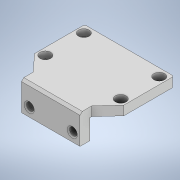
# Autodesk Inventor part: Крышка-6
Saved by Autodesk Inventor 2022 (Build 260153000, 153)
## iProperties
Created: 2021-12-03
Part Number: Крышка-6
Material: Типовые
Document SubType Name: Modeling
Designer: Украинцев
Density: 1 g/cm^3
Appearance: По умолчанию
Author: Украинцев
Autodesk Inventor part; units mm, degrees
ref_plane "YZ Plane" through (0, 0, 0) normal (1, 0, 0) x (0, 1, 0)
ref_plane "XZ Plane" through (0, 0, 0) normal (0, 1, 0) x (-1, 0, 0)
ref_plane "XY Plane" through (0, 0, 0) normal (0, 0, 1) x (1, 0, 0)
sketch "Эскиз1" plane through (0, 0, 0) normal (0, 1, 0) x (-1, 0, 0)
  line L0 (0, 0) -> (58, 0)
  line L1 (58, 0) -> (58, 65)
  line L2 (58, 65) -> (38, 86.8785)
  line L3 (0, 0) -> (0, 102)
  line L4 (0, 102) -> (38, 102)
  line L5 (38, 102) -> (38, 86.8785)
  line L6 (0, 0) -> (49, 0)
  line L7 (49, 0) -> (49, 10)
  line L8 (49, 10) -> (49, 60)
  dimension "d8" = 58
  dimension "d9" = 65
  dimension "d10" = 102
  dimension "d11" = 38
  dimension "d12" = 49
  dimension "d13" = 10
  dimension "d14" = 50
  constraints: 18 end point, 4 perpendicular, 2 coincident, 2 point on line, 1 horizontal, 1 vertical
  measures "d8" distance of L0.start L0.end
  measures "d9" distance of L0.end L1.end
  measures "d10" distance of L0.start L3.end
  measures "d11" distance of L3.end L4.end
  measures "d12" distance of L0.start L6.end
  measures "d13" distance of L6.end L7.end
  measures "d14" distance of L7.end L8.end
extrude "Выдавливание1" add sketch "Эскиз1" along normal blind 12
sketch "Эскиз3" plane through (0, 12, 0) normal (0, 1, 0) x (1, 0, 0)
  line L0 (-38, -102) -> (0, -102) projected
  line L1 (-38, -102) -> (-38, -89)
  line L2 (-38, -86.8785) -> (-38, -102) projected
  line L3 (-38, -89) -> (0, -89)
  line L4 (0, -89) -> (0, -102)
  point P0 (0, 0)
  dimension "d17" = 13
  constraints: 6 end point, 1 perpendicular, 1 point on line, 1 vertical
  measures "d17" distance of L0.start L1.end
extrude "Выдавливание2" add sketch "Эскиз3" against normal blind 38
sketch "Эскиз4" plane through (0, 12, 0) normal (0, 1, 0) x (1, 0, 0)
  line L0 (0, 0) -> (-58, 0) projected
  line L1 (0, 0) -> (-49, 0)
  line L2 (-49, 0) -> (-49, -10)
  line L3 (-49, -10) -> (-49, -60)
  dimension "d20" = 49
  dimension "d21" = 10
  dimension "d22" = 50
  constraints: 6 end point, 2 coincident, 2 point on line, 1 perpendicular
  measures "d20" distance of L0.start L1.end
  measures "d21" distance of L1.end L2.end
  measures "d22" distance of L2.end L3.end
hole "Отверстие1" at (-49, 12, 60) at (-49, 12, 10) direction (0, -1, 0) diameter 9 end through all counterbore diameter 14 counterbore depth 9
sketch "Эскиз6" plane through (-38, 12, 102) normal (0, 0, 1) x (1, 0, 0)
  line L0 (38, -37.7549) -> (10.0011, -38)
  line L1 (0, -38) -> (38, -38) projected
  line L2 (10.0011, -38) -> (10.0011, -27)
  point P0 (38, -12)
  dimension "d39" = 28
  dimension "d40" = 11
  constraints: 4 end point, 1 coincident, 1 point on line, 1 vertical
  measures "d39" distance of L0.start L0.end
  measures "d40" distance of L0.end L2.end
hole "Отверстие3" at (-27.9989, -15, 102) direction (0, 0, -1) diameter 10 end through all
mirror "Зеркальное отражение1" about plane through (0, 0, 102) normal (1, 0, 0) of "Выдавливание2", "Выдавливание1", "Отверстие1", "Отверстие3"
thread "Резьба1" size "M10x1.5" class "6H" standard "ANSI Metric M Profile" full length
thread "Резьба2" size "M10x1.5" class "6H" standard "ANSI Metric M Profile" full length
chamfer "Фаска1" distance 1.6 angle 45 2 edges at (27.9989, -10, 102) (-27.9989, -10, 102)
chamfer "Фаска2" distance 3 angle 45 1 edges at (0, 12, 102)
chamfer "Фаска3" distance 2 angle 45 2 edges at (58, 6, 0) (-58, 6, 0)
